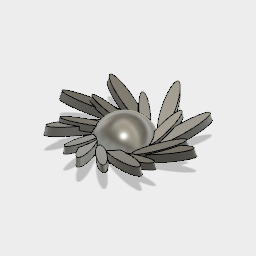
FPROJ_5_Czw (Autodesk Fusion 360 design; units mm, degrees)
Autodesk Fusion 360 part; units mm, degrees
note: some values were not read from the file. Chosen so that the rebuilt part matches the saved one: which bodies a step acts on; which face or edge a step refers to.
sketch "草图1" plane through (0, 0, 0) normal (0, 1, 0) x (1, 0, 0)
  ellipse E0 centre (0, 0) end of major axis (10, 0) minor radius 2
  line L0 (-10, 0) -> (10, 0)
  line L1 (0, -2) -> (0, 2)
extrude "拉伸1" add sketch "草图1" along normal blind 3 makes body 1
move_body "移动1" bodies 1 to x (0.965926, 0, 0.258819) y (0, 1, 0) z (-0.258819, 0, 0.965926) at (0, 0, 0)
box "长方体基本要素1" add length 10 width 10 height 5 placed x (0, 0, 1) y (1, 0, 0) z (0, 1, 0) at (15, 0, 0) separate body makes body 2
move_body "移动2" bodies 1 to x (1, 0, 0) y (0, 1, 0) z (0, 0, 1) at (0.6487, 2.562, -1.5294)
move_body "移动3" bodies 2 to x (1, 0, 0) y (0, 1, 0) z (0, 0, 1) at (10, 5, 15)
move_body "移动4" bodies 1 to x (0.965926, -0.258819, 0) y (0.258819, 0.965926, 0) z (0, 0, 1) at (-1.4174, 0.3574, 0)
move_body "移动5" bodies 2 to x (1, 0, 0) y (0, 1, 0) z (0, 0, 1) at (-15, 0, -5)
pattern_circular "C-阵列1" count 8 over 360 about axis through (10, 10, 10) along (0, -1, 0) of bodies 1 makes body 3 at (11.4128, 4.2387, -8.5815) makes body 4 at (24.1383, 5.2048, -1.8821) makes body 5 at (27.1192, 4.81, 12.3991) makes body 6 at (21.8821, 5.2048, 24.1383) makes body 7 at (7.6009, 4.81, 27.1192) makes body 8 at (-3.8017, 3.8443, 20.6682) makes body 9 at (-8.5815, 4.2387, 8.5872)
copy_body "复制和粘贴实体1" bodies 5 4 9 3 7 6 1 8 makes body 10 makes body 11 makes body 12 makes body 13 makes body 14 makes body 15 makes body 16 makes body 17
scale "缩放1" factor 0.8 about (28.6814, 8.062, 24.1176) bodies 11 15 12 16 17 14 10 13
move_body "移动6" bodies 16 12 10 14 15 11 17 13 to x (0.906308, 0, 0.422618) y (0, 1, 0) z (-0.422618, 0, 0.906308) at (5.1631, 0, -3.2893)
sphere "球体基本要素1" add diameter 20 placed x (1, 0, 0) y (0, 0, -1) z (0, 1, 0) at (47.3228, 0, 16.4497) separate body makes body 18
move_body "MoveFace1" bodies 18 to x (1, 0, 0) y (0, 1, 0) z (0, 0, 1) at (-37, 0, -5) on bodies 18
combine "合并1" operation add target body 1 tool bodies 9 3 4 5 6 7 8 10 11 12 13 14 15 16 17 18 makes body 19 at (19.8036, -2.1279, 9.0859)
box "长方体基本要素2" cut length 195 width 65 height -10 placed x (0, 0, -1) y (-1, 0, 0) z (0, 1, 0) at (50, 0, 120) bodies 19
move_body "移动7" bodies 1 to x (1, 0, 0) y (0, 1, 0) z (0, 0, 1) at (-0.4939, 0, 2.052)
combine "合并2" operation add target body 19 tool bodies 1
hidden bodies 2
